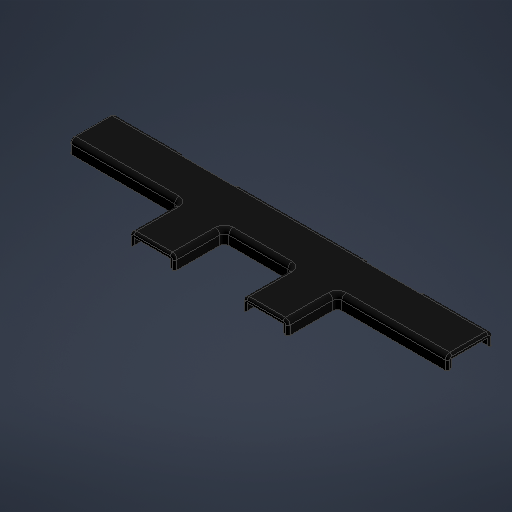
# Autodesk Inventor part: Spiegelflächenabdeckung
Saved by Autodesk Inventor 2025.2 (Build 292293000, 293)
## iProperties
Created: 2025-04-24
Part Number: Spiegelflächenabdeckung
Material: Generisch
Document SubType Name: Modeling
Designer: Faabs
Density: 1 g/cm^3
Appearance: Vorgabe
Author: Faabs
Autodesk Inventor part; units mm, degrees
ref_plane "YZ Plane" through (0, 0, 0) normal (1, 0, 0) x (0, 1, 0)
ref_plane "XZ Plane" through (0, 0, 0) normal (0, 1, 0) x (-1, 0, 0)
ref_plane "XY Plane" through (0, 0, 0) normal (0, 0, 1) x (1, 0, 0)
sketch "Skizze1" plane through (0, 0, 0) normal (0, 0, 1) x (1, 0, 0)
  arc A0 (8.55, -6) -> (6.55, -4) centre (6.55, -6) ccw
  line L0 (6.55, -4) -> (-6.55, -4)
  arc A1 (-6.55, -4) -> (-8.55, -6) centre (-6.55, -6) ccw
  line L1 (-8.55, -6) -> (-8.55, -16)
  line L2 (8.55, -16) -> (8.55, -6)
  arc A2 (-16.55, -6) -> (-18.55, -4) centre (-18.55, -6) ccw
  line L3 (-18.55, -4) -> (-42, -4)
  line L4 (-42, 4) -> (-26.55, 4)
  line L5 (-14.55, 4) -> (14.55, 4)
  line L6 (26.55, 4) -> (42, 4)
  line L7 (42, -4) -> (18.55, -4)
  arc A3 (18.55, -4) -> (16.55, -6) centre (18.55, -6) ccw
  line L8 (16.55, -6) -> (16.55, -16)
  line L9 (-16.55, -16) -> (-16.55, -6)
  line L10 (-26.55, 4) -> (-14.55, 4)
  line L11 (14.55, 4) -> (26.55, 4)
  line L12 (-16.55, -16) -> (-8.55, -16)
  line L13 (8.55, -16) -> (16.55, -16)
  line L14 (-42, 4) -> (-42, -4)
  line L15 (42, 4) -> (42, -4)
  line L16 (-6.55, -5) -> (6.55, -5)
  arc A4 (7.55, -6) -> (6.55, -5) centre (6.55, -6) ccw
  line L17 (7.55, -6) -> (7.55, -17)
  line L18 (7.55, -17) -> (17.55, -17)
  line L19 (17.55, -17) -> (17.55, -6)
  arc A5 (18.55, -5) -> (17.55, -6) centre (18.55, -6) ccw
  line L20 (18.55, -5) -> (43, -5)
  line L21 (43, -5) -> (43, 5)
  line L22 (43, 5) -> (26.55, 5)
  line L23 (26.55, 5) -> (14.55, 5)
  line L24 (14.55, 5) -> (-14.55, 5)
  line L25 (-14.55, 5) -> (-26.55, 5)
  line L26 (-26.55, 5) -> (-43, 5)
  line L27 (-43, 5) -> (-43, -5)
  line L28 (-43, -5) -> (-18.55, -5)
  arc A6 (-17.55, -6) -> (-18.55, -5) centre (-18.55, -6) ccw
  line L29 (-17.55, -6) -> (-17.55, -17)
  line L30 (-17.55, -17) -> (-7.55, -17)
  line L31 (-7.55, -17) -> (-7.55, -6)
  arc A7 (-6.55, -5) -> (-7.55, -6) centre (-6.55, -6) ccw
  line L32 (-42, 5) -> (-42, -5)
  line L33 (42, 5) -> (42, -5)
  line L34 (17.55, -16) -> (-17.55, -16)
  line L35 (-6.55, -3.9) -> (6.55, -3.9)
  arc A8 (8.65, -6) -> (6.55, -3.9) centre (6.55, -6) ccw
  line L36 (8.65, -6) -> (8.65, -15.9)
  line L37 (8.65, -15.9) -> (16.45, -15.9)
  line L38 (16.45, -15.9) -> (16.45, -6)
  arc A9 (18.55, -3.9) -> (16.45, -6) centre (18.55, -6) ccw
  line L39 (18.55, -3.9) -> (41.9, -3.9)
  line L40 (41.9, -3.9) -> (41.9, 3.9)
  line L41 (41.9, 3.9) -> (26.55, 3.9)
  line L42 (26.55, 3.9) -> (14.55, 3.9)
  line L43 (14.55, 3.9) -> (-14.55, 3.9)
  line L44 (-14.55, 3.9) -> (-26.55, 3.9)
  line L45 (-26.55, 3.9) -> (-41.9, 3.9)
  line L46 (-41.9, 3.9) -> (-41.9, -3.9)
  line L47 (-41.9, -3.9) -> (-18.55, -3.9)
  arc A10 (-16.45, -6) -> (-18.55, -3.9) centre (-18.55, -6) ccw
  line L48 (-16.45, -6) -> (-16.45, -15.9)
  line L49 (-16.45, -15.9) -> (-8.65, -15.9)
  line L50 (-8.65, -15.9) -> (-8.65, -6)
  arc A11 (-6.55, -3.9) -> (-8.65, -6) centre (-6.55, -6) ccw
  line L51 (0, 0) -> (-20.55, 0)
  line L52 (-20.55, 0) -> (-20.55, 3.9)
  point P0 (-16.55, -16)
  point P1 (16.55, -16)
  point P2 (-8.55, -16)
  point P3 (-7.55, -16)
  point P4 (7.55, -16)
  point P5 (8.55, -16)
  dimension "d0" = 1
  dimension "d1" = 0.1
  dimension "d12" = 20.55
  constraints: 106 end point, 24 point on circle, 12 centre point, 12 perpendicular, 9 point on line, 3 collinear, 2 horizontal, 1 midpoint, 38 other
  measures "d0" distance between parallel lines of L0 L16
  measures "d1" distance between parallel lines of L0 L35
  measures "d12" distance of L51.start L51.end
extrude "Extrusion1" add sketch "Skizze1" against normal blind 1 contours A0 L0 A1 L1 L12 L9 A2 L3 L14 L4 L10 L5 L11 L6 L15 L7 A3 L8 L13 L2 | A11 L50 L49 L48 A10 L47 L46 L45 L44 L43 L42 L41 L40 L39 A9 L38 L37 L36 A8 L35
extrude "Extrusion2" add sketch "Skizze1" against normal blind 3 contours L2 L34 L17 A4 L16 A7 L31 L1 A1 L0 A0 | L8 A3 L7 L33 L20 A5 L19 L34 | L34 L29 A6 L28 L32 L3 A2 L9 | L6 L11 L5 L10 L4 L32 L26 L25 L24 L23 L22 L33
fillet "Rundung1" radius 1 12 edges at (-17.8429, -5.2929, 0) (-30.275, -5, 0) (-17.55, -11, 0) (-7.2571, -5.2929, 0) (0, -5, 0) (7.2571, -5.2929, 0) (7.55, -11, 0) (-7.55, -11, 0) (17.8429, -5.2929, 0) (17.55, -11, 0) (30.275, -5, 0) (0, 5, 0)
chamfer "Fasen1" distance 0.5 angle 45 12 edges at (-16.55, -11, -3) (-17.1358, -4.5858, -3) (-30.275, -4, -3) (-8.55, -11, -3) (-7.9642, -4.5858, -3) (0, -4, -3) (7.9642, -4.5858, -3) (8.55, -11, -3) (17.1358, -4.5858, -3) (30.275, -4, -3) (16.55, -11, -3) (0, 4, -3)
fillet "Rundung2" radius 0.5 20 edges at (-42, -4.7071, -0.2929) (-42, 0, 0) (-42, 4.7071, -0.2929) (-42, 5, -2) (-42, -5, -2) (-7.8429, -16, -0.2929) (-7.55, -16, -2) (-17.2571, -16, -0.2929) (-17.55, -16, -2) (-12.55, -16, 0) (17.2571, -16, -0.2929) (17.55, -16, -2) (7.8429, -16, -0.2929) (7.55, -16, -2) (12.55, -16, 0) (42, 4.7071, -0.2929) (42, 5, -2) (42, -4.7071, -0.2929) (42, -5, -2) (42, 0, 0)
sketch "Skizze2" plane through (0, 0, 0) normal (0, 0, 1) x (1, 0, 0)
  circle A0 centre (20.55, 8) radius 1.2295
  circle A1 centre (-20.55, 8) radius 1.2295
  arc A2 (8.55, -6) -> (6.55, -4) centre (6.55, -6) ccw
  line L0 (6.55, -4) -> (-6.55, -4)
  arc A3 (-6.55, -4) -> (-8.55, -6) centre (-6.55, -6) ccw
  line L1 (-8.55, -6) -> (-8.55, -23)
  line L2 (8.55, -23) -> (8.55, -6)
  arc A4 (-16.55, -6) -> (-18.55, -4) centre (-18.55, -6) ccw
  line L3 (-18.55, -4) -> (-46, -4)
  arc A5 (-46, 4) -> (-46, -4) centre (-46, 0) ccw
  line L4 (-46, 4) -> (-26.55, 4)
  arc A6 (-26.55, 4) -> (-24.55, 6) centre (-26.55, 6) ccw
  line L5 (-24.55, 6) -> (-24.55, 8)
  arc A7 (-16.55, 8) -> (-24.55, 8) centre (-20.55, 8) ccw
  line L6 (-16.55, 8) -> (-16.55, 6)
  arc A8 (-16.55, 6) -> (-14.55, 4) centre (-14.55, 6) ccw
  line L7 (-14.55, 4) -> (14.55, 4)
  arc A9 (14.55, 4) -> (16.55, 6) centre (14.55, 6) ccw
  line L8 (16.55, 6) -> (16.55, 8)
  arc A10 (24.55, 8) -> (16.55, 8) centre (20.55, 8) ccw
  line L9 (24.55, 8) -> (24.55, 6)
  arc A11 (24.55, 6) -> (26.55, 4) centre (26.55, 6) ccw
  line L10 (26.55, 4) -> (46, 4)
  arc A12 (46, -4) -> (46, 4) centre (46, 0) ccw
  line L11 (46, -4) -> (18.55, -4)
  arc A13 (18.55, -4) -> (16.55, -6) centre (18.55, -6) ccw
  line L12 (16.55, -6) -> (16.6007, -43)
  line L13 (-16.5067, -43) -> (-16.55, -6)
  circle A14 centre (46, 0) radius 1.45
  circle A15 centre (-46, 0) radius 1.45
  line L14 (0, 4) -> (0, -4)
  line L15 (16.8007, -42.9997) -> (16.75, -6.0025)
  arc A16 (18.55, -4.2) -> (16.75, -6.0025) centre (18.55, -6) ccw
  line L16 (18.55, -4.2) -> (46, -4.2)
  arc A17 (46, -4.2) -> (46, 4.2) centre (46, 0) ccw
  line L17 (46, 4.2) -> (26.55, 4.2)
  arc A18 (24.75, 6) -> (26.55, 4.2) centre (26.55, 6) ccw
  line L18 (24.75, 6) -> (24.75, 8)
  arc A19 (24.75, 8) -> (16.35, 8) centre (20.55, 8) ccw
  line L19 (16.35, 8) -> (16.35, 6)
  arc A20 (14.55, 4.2) -> (16.35, 6) centre (14.55, 6) ccw
  line L20 (14.55, 4.2) -> (-14.55, 4.2)
  arc A21 (-16.35, 6) -> (-14.55, 4.2) centre (-14.55, 6) ccw
  line L21 (-16.35, 6) -> (-16.35, 8)
  arc A22 (-16.35, 8) -> (-24.75, 8) centre (-20.55, 8) ccw
  line L22 (-24.75, 8) -> (-24.75, 6)
  arc A23 (-26.55, 4.2) -> (-24.75, 6) centre (-26.55, 6) ccw
  line L23 (-26.55, 4.2) -> (-46, 4.2)
  arc A24 (-46, 4.2) -> (-46, -4.2) centre (-46, 0) ccw
  line L24 (-46, -4.2) -> (-18.55, -4.2)
  arc A25 (-16.75, -5.9957) -> (-18.55, -4.2) centre (-18.55, -6) ccw
  line L25 (-16.75, -5.9957) -> (-16.7067, -43.0002)
  line L26 (41.5, 5) -> (-41.5, 5) projected
  line L27 (-26.55, 5) -> (-26.55, 4)
  line L28 (-14.55, 4.2) -> (-14.55, 5)
  line L29 (-14.55, 4.2) -> (-14.55, 4)
  line L30 (14.55, 4.2) -> (14.55, 5)
  line L31 (14.55, 4.2) -> (14.55, 4)
  line L32 (26.55, 4.2) -> (26.55, 5)
  line L33 (26.55, 4.2) -> (26.55, 4)
  line L34 (14.55, 4) -> (26.55, 4)
  line L35 (-26.55, 4) -> (-20.55, 4)
  line L36 (-41.5, 4) -> (41.5, 4) projected
  line L37 (-20.55, 4) -> (-14.55, 4)
  line L38 (-26.55, 5) -> (-14.55, 5)
  line L39 (14.55, 5) -> (26.55, 5)
  point P0 (0, 0)
  point P1 (0, 0)
  dimension "d13" = 0.2
  constraints: 76 end point, 44 point on circle, 26 centre point, 6 collinear, 5 point on line, 4 perpendicular, 3 midpoint, 1 vertical, 20 other
  measures "d13" radial gap between concentric circles of A6 A23
extrude "Extrusion3" cut sketch "Skizze2" against normal blind 3 contours L27 A23 L26 A6 | A6 L26 A8 L36 L35 | L27 L26 A23 | L26 A21 L29 A8 | L26 L28 A21 | L31 A20 L26 A9 | A9 L26 A11 L34 | L30 L26 A20 | A11 L26 A18 L33 | A18 L26 L32
fillet "Rundung3" radius 0.5 11 edges at (26.55, 5, -2) (26.55, 4.7746, -0.3675) (26.55, 4.1005, -0.0051) (14.55, 4.1005, -0.0051) (14.55, 4.7746, -0.3675) (14.55, 5, -2) (-26.55, 4.7071, -0.2929) (-26.55, 5, -2) (-14.55, 5, -2) (-14.55, 4.7746, -0.3675) (-14.55, 4.1005, -0.0051)
